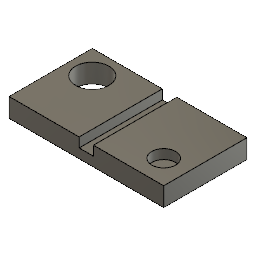
CAM Test v3 (Autodesk Fusion 360 design; units mm, degrees)
Autodesk Fusion 360 part; units mm, degrees
sketch "Sketch1" plane through (0, 0, 0) normal (0, 1, 0) x (1, 0, 0)
  line L0 (0, 0) -> (65, 0)
  line L1 (65, 0) -> (65, 35)
  line L2 (65, 35) -> (0, 35)
  line L3 (0, 35) -> (0, 0)
  line L4 (10, 35) -> (10, 25) construction
  circle A0 centre (10, 25) radius 7
  dimension "d1" = 35
  dimension "d2" = 65
  dimension "d3" = 14
  measures "d3" diameter of A0
extrude "Extrude1" add sketch "Sketch1" along normal blind 8
sketch "Sketch2" plane through (0, 8, 0) normal (0, 1, 0) x (-1, 0, 0)
  circle A0 centre (-10, -25) radius 7
  line L0 (0, -35) -> (0, 0)
  line L1 (0, 0) -> (-65, 0)
  line L2 (-65, 0) -> (-65, -35)
  line L3 (-65, -35) -> (0, -35)
  circle A1 centre (-55, -10) radius 5
  dimension "d6" = 10
  measures "d6" diameter of A1
extrude "Extrude2" cut sketch "Sketch2" against normal blind 4 contours A1
sketch "Sketch3" plane through (0, 0, 0) normal (0, 0, 1) x (1, 0, 0)
  line L0 (0, 0) -> (65, 0)
  line L1 (65, 0) -> (65, 8)
  line L2 (65, 8) -> (0, 8)
  line L3 (0, 8) -> (0, 0)
  line L4 (32.5, 8) -> (35.5, 8)
  line L5 (35.5, 8) -> (35.5, 4)
  line L6 (35.5, 4) -> (29.5, 4)
  line L7 (29.5, 4) -> (29.4914, 8)
  line L8 (32.5, 8) -> (29.4914, 8)
  dimension "d9" = 3
  dimension "d10" = 4
  dimension "d11" = 6
extrude "Extrude3" cut sketch "Sketch3" against normal blind 35 contours L2 L4 L5 L6 L7 L8
